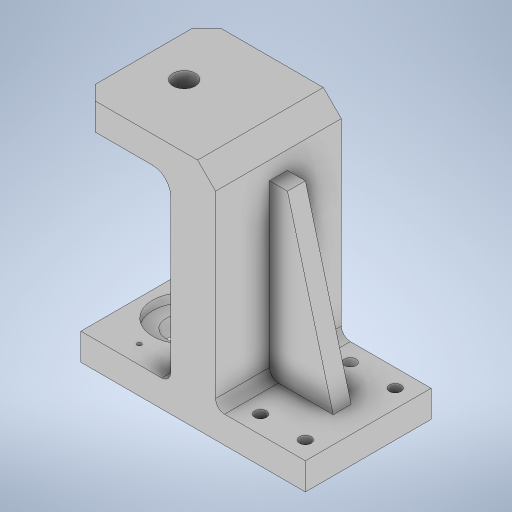
# Autodesk Inventor part: Base do Amassador
Saved by Autodesk Inventor 2023 (Build 270158030, 158C)
## iProperties
Created: 2022-07-17
Part Number: Base do Amassador
Material: Generic
Document SubType Name: Modeling
Designer: coqui
Density: 1 g/cm^3
Appearance: Default
Author: coqui
Autodesk Inventor part; units mm, degrees
ref_plane "YZ Plane" through (0, 0, 0) normal (1, 0, 0) x (0, 1, 0)
ref_plane "XZ Plane" through (0, 0, 0) normal (0, 1, 0) x (-1, 0, 0)
ref_plane "XY Plane" through (0, 0, 0) normal (0, 0, 1) x (1, 0, 0)
sketch "Sketch1" plane through (0, 0, 0) normal (0, 0, 1) x (1, 0, 0)
  line L0 (-126.8193, 0) -> (-126.8193, 30)
  line L1 (-126.8193, 30) -> (-36.8193, 30)
  line L2 (-26.8193, 40) -> (-26.8193, 210)
  line L3 (-46.8193, 230) -> (-126.8193, 230)
  line L4 (-126.8193, 230) -> (-126.8193, 260)
  line L5 (-126.8193, 260) -> (3.1807, 260)
  line L6 (23.1807, 240) -> (23.1807, 40)
  line L7 (33.1807, 30) -> (123.1807, 30)
  line L8 (123.1807, 30) -> (123.1807, 0)
  line L9 (-126.8193, 0) -> (123.1807, 0)
  line L10 (3.1807, 260) -> (23.1807, 240)
  arc A0 (-36.8193, 30) -> (-26.8193, 40) centre (-36.8193, 40) ccw
  arc A1 (23.1807, 40) -> (33.1807, 30) centre (33.1807, 40) ccw
  arc A2 (-26.8193, 210) -> (-46.8193, 230) centre (-46.8193, 210) ccw
  point P0 (0, 0)
  point P1 (-26.8193, 30)
  point P2 (-26.8193, 230)
  point P3 (23.1807, 260)
  point P4 (23.1807, 30)
  dimension "d0" = 250
  dimension "d1" = 100
  dimension "d2" = 100
  dimension "d3" = 100
  dimension "d4" = 50
  dimension "d5" = 30
  dimension "d7" = 200
  dimension "d8" = 260
  dimension "d9" = 150
  dimension "d10" = 20
  dimension "d11" = 20
  dimension "d12" = 10
  dimension "d13" = 20
  constraints: 22 end point, 10 point on line, 7 perpendicular, 6 point on circle, 6 tangent, 3 centre point, 1 equal radius, 1 horizontal
  measures "d0" distance of L8.end L0.start
  measures "d1" distance of L0.end point (-26.819, 30)
  measures "d2" distance of point (23.181, 30) L7.end
  measures "d3" distance of point (-26.819, 230) L3.end
  measures "d4" distance between parallel lines of L6 L2
  measures "d5" distance of L8.end L7.end
  measures "d7" distance of point (-26.819, 30) point (-26.819, 230)
  measures "d8" distance of L0.start L4.end
  measures "d9" distance of L4.end point (23.181, 260)
  measures "d10" distance of L5.end point (23.181, 260)
  measures "d11" distance of L6.start point (23.181, 260)
  measures "d12" radius of A0
  measures "d13" radius of A2
extrude "Extrusion1" add sketch "Sketch1" along normal mid plane 140
chamfer "Chamfer1" distance 16 angle 45 2 edges at (-126.8193, 245, 70) (-126.8193, 245, -70)
sketch "Sketch2" plane through (0, 0, 0) normal (0, 0, 1) x (1, 0, 0)
  line L0 (23.1807, 240) -> (23.1807, 40) projected
  line L1 (23.1807, 220) -> (43.1807, 220)
  line L2 (43.1807, 220) -> (94.0911, 30)
  line L3 (123.1807, 30) -> (33.1807, 30) projected
  point P0 (0, 0)
  dimension "d19" = 20
  dimension "d20" = 190
  dimension "d22" = 15
  constraints: 4 end point, 2 point on line, 1 perpendicular
  measures "d19" distance of L1.start L1.end
  measures "d20" vertical distance of L1.end L2.end
  measures "d22" angle of L0 L2
extrude "Rib1" add sketch "Sketch2" along normal mid plane 20 rib yes fills toward (33.1807, 219.95) open curves L1 L2
sketch "Sketch3" plane through (-126.8193, 30, 70) normal (0, 1, 0) x (1, 0, 0)
  circle A0 centre (45, 70) radius 35
  line L0 (0, 124) -> (0, 16) projected
  point P0 (126.8193, 70)
  dimension "d30" = 45
  dimension "d31" = 70
  constraints: 1 centre point
  measures "d30" distance from line of L0 A0.centre
  measures "d31" diameter of A0
extrude "Extrusion2" cut sketch "Sketch3" against normal blind 10
sketch "Sketch4" plane through (-81.8193, 20, 0) normal (0, 1, 0) x (1, 0, 0)
  circle A0 centre (0, 0) radius 35 projected
  circle A1 centre (0, 0) radius 20
  point P0 (81.8193, 0)
  dimension "d34" = 40
  constraints: 1 centre point, 1 coincident
  measures "d34" diameter of A1
extrude "Extrusion3" cut sketch "Sketch4" against normal blind 20 contours A1
sketch "Sketch5" plane through (3.1807, 260, 70) normal (0, 1, 0) x (1, 0, 0)
  circle A0 centre (-85, 70) radius 12.5
  point P0 (-3.1807, 70)
  dimension "d37" = 25
  constraints: 1 centre point, 1 coincident
  measures "d37" diameter of A0
extrude "Extrusion4" cut sketch "Sketch5" against normal through all
sketch "Sketch6" plane through (-126.8193, 30, 70) normal (0, 1, 0) x (1, 0, 0)
  circle A0 centre (45, 20) radius 2.46
  circle A1 centre (45, 120) radius 2.46
  circle A2 centre (45, 70) radius 12.5 projected
  point P0 (126.8193, 70)
  dimension "d40" = 4.92
  dimension "d41" = 100
  dimension "d42" = 4.92
  dimension "d43" = 50
  dimension "d44" = 50
  constraints: 2 centre point
  measures "d40" diameter of A0
  measures "d41" distance of A1.centre A0.centre
  measures "d42" diameter of A1
  measures "d43" distance of A2.centre A0.centre
  measures "d44" distance of A1.centre A2.centre
extrude "Extrusion5" cut sketch "Sketch6" against normal blind 30 contours A0 | A1
sketch "Sketch7" plane through (33.1807, 30, 70) normal (0, 1, 0) x (1, 0, 0)
  circle A0 centre (20, 120) radius 6.5
  line L0 (90, 140) -> (90, 0) projected
  line L1 (0, 140) -> (90, 140) projected
  circle A1 centre (70, 120) radius 6.5
  circle A2 centre (20, 20) radius 6.5
  circle A3 centre (70, 20) radius 6.5
  point P0 (-33.1807, 70)
  dimension "d47" = 13
  dimension "d48" = 70
  dimension "d49" = 20
  dimension "d52" = 50
  dimension "d55" = 100
  constraints: 4 centre point, 1 horizontal, 1 vertical, 6 other
  measures "d47" diameter of A0
  measures "d48" distance from line of L0 A0.centre
  measures "d49" distance from line of L1 A0.centre
  measures "d52" distance of A0.centre A1.centre
  measures "d55" distance of A0.centre A2.centre
extrude "Extrusion6" cut sketch "Sketch7" against normal blind 30
equation "\"d11\" = d10"
body "Solid1"
